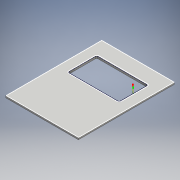
# Autodesk Inventor part: masca raspberry
Saved by Autodesk Inventor 2016 (Build 200138000, 138)
## iProperties
Created: 2016-02-21
Part Number: masca raspberry
Material: Generic
Document SubType Name: Modeling
Designer: roduino
Density: 1 g/cm^3
Appearance: Default
Author: roduino
Autodesk Inventor part; units mm, degrees
ref_plane "YZ Plane" through (0, 0, 0) normal (1, 0, 0) x (0, 1, 0)
ref_plane "XZ Plane" through (0, 0, 0) normal (0, 1, 0) x (-1, 0, 0)
ref_plane "XY Plane" through (0, 0, 0) normal (0, 0, 1) x (1, 0, 0)
sketch "Sketch1" plane through (0, 0, 0) normal (0, 0, 1) x (1, 0, 0)
  line L0 (-132.5, 175) -> (132.5, 175)
  line L1 (132.5, 175) -> (132.5, -175)
  line L2 (132.5, -175) -> (-132.5, -175)
  line L3 (-132.5, -175) -> (-132.5, 175)
  point P0 (0, 0)
  dimension "d0" = 265
  dimension "d1" = 350
  dimension "d2" = 265
  dimension "d3" = 350
  dimension "d4" = 132.5
  dimension "d5" = 175
  constraints: 8 end point, 2 parallel, 1 horizontal, 1 perpendicular
  measures "d0" distance of L1.end L2.end
  measures "d1" distance of L0.end L1.end
  measures "d2" distance of L0.start L0.end
  measures "d3" distance of L2.end L0.start
  measures "d4" distance from line of point (0, 0) L3
  measures "d5" distance from line of point (0, 0) L0
extrude "Extrusion1" add sketch "Sketch1" along normal blind 8
sketch "Sketch2" plane through (0, 0, 8) normal (0, 0, 1) x (1, 0, 0)
  line L0 (-96.5, 121) -> (96.5, 121)
  line L1 (96.5, 121) -> (96.5, 10)
  line L2 (96.5, 10) -> (-96.5, 10)
  line L3 (-96.5, 10) -> (-96.5, 121)
  point P0 (0, 0)
  dimension "d8" = 193
  dimension "d9" = 111
  dimension "d10" = 96.5
  dimension "d17" = 10
  constraints: 8 end point, 2 parallel, 1 horizontal, 1 perpendicular
  measures "d8" distance of L0.start L0.end
  measures "d9" distance of L2.end L0.start
  measures "d10" distance from line of point (0, 0) L3
  measures "d17" distance from line of point (0, 0) L2
extrude "Extrusion2" cut sketch "Sketch2" against normal blind 1
fillet "Fillet1" radius 8 4 edges at (-96.5, 121, 7.5) (96.5, 121, 7.5) (96.5, 10, 7.5) (-96.5, 10, 7.5)
sketch "Sketch3" plane through (0, 0, 7) normal (0, 0, 1) x (1, 0, 0)
  arc A0 (-96.5, 18) -> (-88.5, 10) centre (-88.5, 18) ccw projected
  line L0 (88.5, 10) -> (-88.5, 10) projected
  arc A1 (88.5, 10) -> (96.5, 18) centre (88.5, 18) ccw projected
  line L1 (96.5, 113) -> (96.5, 18) projected
  arc A2 (96.5, 113) -> (88.5, 121) centre (88.5, 113) ccw projected
  line L2 (-88.5, 121) -> (88.5, 121) projected
  arc A3 (-88.5, 121) -> (-96.5, 113) centre (-88.5, 113) ccw projected
  line L3 (-96.5, 18) -> (-96.5, 113) projected
  arc A4 (-88.5, 117.5) -> (-93, 113) centre (-88.5, 113) ccw
  line L4 (-88.5, 117.5) -> (88.5, 117.5)
  arc A5 (93, 113) -> (88.5, 117.5) centre (88.5, 113) ccw
  line L5 (93, 113) -> (93, 18)
  arc A6 (88.5, 13.5) -> (93, 18) centre (88.5, 18) ccw
  line L6 (88.5, 13.5) -> (-88.5, 13.5)
  arc A7 (-93, 18) -> (-88.5, 13.5) centre (-88.5, 18) ccw
  line L7 (-93, 18) -> (-93, 113)
  point P0 (0, 0)
  dimension "d14" = 3.5
  constraints: 8 end point, 8 point on circle, 4 centre point, 7 other
  measures "d14" distance between parallel lines of L3 L7
extrude "Extrusion3" cut sketch "Sketch3" against normal through all contours L4 A5 L5 A6 L6 A7 L7 A4
equation "\"d4\" = 0.5 * d2"
equation "\"d5\" = 0.5 * d3"
equation "\"d10\" = 0.5 * d8"
body "Solid1"
